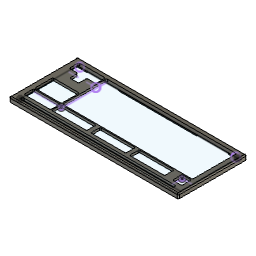
TKL assembled v2 (Autodesk Fusion 360 archive; units mm, degrees)
design "top attempt"
Autodesk Fusion 360 part; units mm, degrees
note: some values were not read from the file. Chosen so that the rebuilt part matches the saved one: which face or edge a step refers to. Set by a fixed rule: which sketch regions a step uses.
sketch "Sketch1" plane through (0, 0, 0) normal (1, 0, 0) x (0, 1, 0)
  line L0 (70, 20) -> (-80, 20)
  line L1 (-80, 20) -> (-80, 10)
  line L2 (-80, 10) -> (70, 10)
  line L3 (70, 10) -> (70, 20)
  constraint horizontal L0
  constraint vertical L1
  constraint horizontal L2
  constraint vertical L3
extrude "Extrude1" add sketch "Sketch1" along normal blind 185
move_face "OffsetFaces1" offset 185 1 faces at (0, -30, 13.3333)
sketch "Sketch2" plane through (0, 0, 20) normal (0, 0, 1) x (-1, 0, 0)
  line L0 (185, -70) -> (185, 80)
  line L1 (185, 80) -> (-185, 80)
  line L2 (-185, 80) -> (-185, -70)
  line L3 (-185, -70) -> (185, -70)
  line L4 (0, 0) -> (-110, 0)
  line L5 (0, 0) -> (175, 0)
  line L6 (0, 70) -> (0, 10)
  line L7 (0, 10) -> (0, -35)
  line L8 (175, 0) -> (175, -35)
  line L9 (175, -35) -> (-110, 70)
  line L10 (-110, -35) -> (-110, 70)
  line L11 (-110, 70) -> (175, 70)
  line L12 (175, 70) -> (175, -35)
  line L13 (-175, 70) -> (-116.5, 70)
  line L14 (-116.5, 70) -> (-116.5, 50.5)
  line L15 (-116.5, 50.5) -> (-175, 50.5)
  line L16 (-175, 50.5) -> (-175, 70)
  line L17 (-175, 50.5) -> (-155.5, 50.5)
  line L18 (-155.5, 50.5) -> (-155.5, 41.913)
  line L19 (-155.5, 50.5) -> (-155.5, 70)
  line L20 (-155.5, 41.913) -> (-136, 41.913)
  line L21 (-155.5, 70) -> (-136, 70)
  line L22 (-136, 70) -> (-136, 31)
  line L23 (-136, 31) -> (-155.5, 31)
  line L24 (-155.5, 31) -> (-155.5, 70)
  line L25 (-90, 70) -> (-90, -25)
  line L26 (-90, -25) -> (-110, -25)
  line L27 (-90, -25) -> (175, -25.0645)
  line L28 (-117.5, -25) -> (-175, -25)
  line L29 (-175, -25) -> (-175, 10)
  line L30 (-175, 10) -> (-117.5, 10)
  line L31 (-117.5, 10) -> (-117.5, -25)
  line L32 (-110, 8.1702) -> (-113, 8.1702)
  dimension "d4" = 110
  dimension "d5" = 175
  dimension "d8" = 60
  dimension "d9" = 45
  dimension "d12" = 19.5
  dimension "d13" = 19.5
  dimension "d14" = 19.5
  dimension "d15" = 39
  dimension "d16" = 95
  constraint coincident L4.start L5.start
  constraint horizontal L4
  constraint parallel L3 L5
  constraint perpendicular L4 L6
  constraint perpendicular L4 L7
  constraint perpendicular L5 L8
  constraint vertical L10
  constraint horizontal L11
  constraint vertical L12
  constraint perpendicular L13 L14
  constraint parallel L13 L15
  constraint parallel L14 L16
  constraint horizontal L13
  constraint horizontal L17
  constraint vertical L18
  constraint coincident L13 L19.end
  constraint perpendicular L13 L19
  constraint perpendicular L18 L20
  constraint horizontal L21
  constraint vertical L22
  constraint horizontal L23
  constraint vertical L24
  constraint coincident L11 L25.start
  constraint perpendicular L4 L25
  constraint coincident L10 L26.end
  constraint perpendicular L10 L26
  constraint coincident L8 L27.end
  constraint horizontal L28
  constraint vertical L29
  constraint horizontal L30
  constraint vertical L31
  constraint coincident L10 L32.start
  constraint perpendicular L31 L32
  measures "d4" distance of L4.start L4.end
  measures "d5" distance of L4.start L5.end
  measures "d8" distance of L6.start L6.end
  measures "d9" distance of L6.end L7.end
  measures "d12" distance of L13.start L15.end
  measures "d13" distance of L15.end L17.end
  measures "d14" distance of L18.end L20.end
  measures "d15" distance of L19.end L23.end
  measures "d16" distance of L25.start L25.end
sketch "Sketch3" plane through (0, 0, 0) normal (0, 0, 1) x (1, 0, 0)
extrude "Extrude2" add sketch "Sketch2" along normal blind 1 contours L28 L29 L30 L31
extrude "Extrude3" cut 1 faces at (136.6667, 13.3333, 21) along direction (0, 0, -1) blind 1
sketch "Sketch4" plane through (0, 0, 20) normal (0, 0, 1) x (-1, 0, 0)
  line L0 (185, -70) -> (185, 80)
  line L1 (185, 80) -> (-185, 80)
  line L2 (-185, 80) -> (-185, -70)
  line L3 (-185, -70) -> (185, -70)
  line L4 (-172.5, 0) -> (-172.5, -60)
  line L5 (172.5, 0) -> (172.5, 60)
  line L6 (-172.5, -60) -> (172.5, -60)
  line L7 (172.5, -60) -> (172.5, 60)
  line L8 (172.5, 60) -> (-172.5, 60)
  line L9 (-172.5, 60) -> (-172.5, -60)
  line L10 (0, -60) -> (0, 36)
  line L11 (-172.5, 36) -> (-172.5, -60)
  line L12 (-172.5, -60) -> (114.5, -60)
  line L13 (-172.5, -60) -> (111.5, -60)
  line L14 (-172.5, -60) -> (111.5, -60)
  line L15 (112, 36.5) -> (-172.5, 36.5)
  line L16 (-172.5, 36.5) -> (-172.5, -60)
  line L17 (172.5, -60) -> (115, -60)
  line L18 (172.5, -41) -> (172.5, -60)
  line L19 (153.5, -41) -> (134, -41)
  line L20 (134, -41) -> (134, -21)
  line L21 (134, -21) -> (153.5, -21)
  line L22 (153.5, -21) -> (153.5, -41)
  line L23 (172.5, 36) -> (172.5, -3)
  line L24 (172.5, 36) -> (172.5, -3)
  line L25 (172.5, -3) -> (112, -3)
  line L26 (-172.5, 60) -> (-152.5, 60)
  line L27 (-172.5, 40) -> (-172.5, 60)
  line L28 (172.5, 60) -> (114.5, 60)
  line L29 (114.5, 60) -> (114.5, 39)
  line L30 (114.5, 39) -> (172.5, 39)
  line L31 (172.5, 39) -> (172.5, 60)
  line L32 (-134.5, 60) -> (-58, 60)
  line L33 (-49, 60) -> (27.5, 60)
  line L34 (112, 39) -> (35.5, 39)
  line L35 (35.5, 39) -> (35.5, 60)
  line L36 (35.5, 60) -> (112, 60)
  line L37 (112, 60) -> (112, 39)
  line L38 (26.5, 55.7624) -> (26.5, 60.0294)
  line L39 (26.5, 60.0294) -> (-50, 60.0294)
  line L40 (-50, 60.0294) -> (-50, 39)
  line L41 (-50, 39) -> (26.5, 39)
  line L42 (26.5, 39) -> (26.5, 60.0294)
  line L43 (-58.5, 51.7468) -> (-58.5, 60)
  line L44 (-58.5, 60) -> (-135, 60)
  line L45 (-135, 60) -> (-135, 39)
  line L46 (-135, 39) -> (-58.5, 39)
  line L47 (-58.5, 39) -> (-58.5, 60)
  line L48 (114.5, -39) -> (172.5, -39)
  line L49 (115, -60) -> (112, -60)
  line L50 (112, -60) -> (112, 36.5)
  line L51 (114, 35) -> (115, 35)
  line L52 (115, 35) -> (114.5, 35)
  line L53 (114.5, 36) -> (114.5, -3)
  line L54 (114.5, -3) -> (114.5, -60)
  line L55 (114.5, 36) -> (114.5, 37)
  line L56 (114.5, 37) -> (114.5, 36.5)
  line L57 (117.4051, 36.5) -> (114.5, 36.5)
  line L58 (117.4051, 36.5) -> (172.5, 36.5)
  line L59 (112, 37) -> (112, 36.5)
  line L60 (-152.5, 60) -> (-152.5, 39)
  line L61 (-152.5, 39) -> (-172.5, 39)
  dimension "d21" = 172.5
  dimension "d22" = 172.5
  dimension "d24" = 96
  dimension "d26" = 284
  dimension "d27" = 57.5
  dimension "d28" = 19
  dimension "d29" = 19
  dimension "d31" = 39
  dimension "d32" = 20
  dimension "d33" = 20
  dimension "d37" = 76.5
  dimension "d39" = 4.267
  dimension "d41" = 76.5
  constraint horizontal L6
  constraint vertical L7
  constraint horizontal L8
  constraint vertical L9
  constraint midpoint L6 L10.start
  constraint vertical L11
  constraint horizontal L12
  constraint perpendicular L4 L13
  constraint horizontal L14
  constraint horizontal L15
  constraint vertical L16
  constraint perpendicular L7 L17
  constraint perpendicular L19 L20
  constraint parallel L19 L21
  constraint parallel L20 L22
  constraint vertical L24
  constraint horizontal L25
  constraint perpendicular L9 L26
  constraint horizontal L28
  constraint vertical L29
  constraint horizontal L30
  constraint vertical L31
  constraint coincident L8 L32.start
  constraint coincident L8 L33.start
  constraint perpendicular L34 L35
  constraint parallel L34 L36
  constraint parallel L35 L37
  constraint vertical L38
  constraint perpendicular L39 L40
  constraint parallel L39 L41
  constraint parallel L40 L42
  constraint perpendicular L38 L39
  constraint vertical L43
  constraint perpendicular L44 L45
  constraint parallel L44 L46
  constraint parallel L45 L47
  constraint coincident L8 L44.end
  constraint coincident L7 L48.end
  constraint perpendicular L7 L48
  constraint coincident L6 L49.end
  constraint perpendicular L15 L50
  constraint coincident L25.end L50
  constraint perpendicular L50 L51
  constraint midpoint L51 L52.end
  constraint parallel L51 L52
  constraint coincident L25 L53.end
  constraint perpendicular L25 L53
  constraint parallel L53 L55
  constraint midpoint L55 L56.end
  constraint parallel L55 L56
  constraint perpendicular L55 L57
  constraint coincident L5 L58.end
  constraint coincident L7 L58.end
  constraint perpendicular L15 L59
  constraint perpendicular L26 L60
  constraint coincident L9 L61.end
  constraint perpendicular L9 L61
  constraint coincident L48.start L54
  measures "d21" distance of origin L4.start
  measures "d22" distance of origin L5.start
  measures "d24" distance of L10.start L10.end
  measures "d26" distance of L4.end L13.end
  measures "d27" distance of L6.end L17.end
  measures "d28" distance of L6.end L18.start
  measures "d29" distance of L18.start L19.start
  measures "d31" distance of L23.start L23.end
  measures "d32" distance of L8.end L26.end
  measures "d33" distance of L8.end L27.start
  measures "d37" distance of L34.start L34.end
  measures "d39" distance of L38.start L38.end
  measures "d41" distance of L43.end L44.end
extrude "Extrude4" cut sketch "Sketch4" against normal blind 20 contours L4 L6 L9 L11 L12 L13 L14 L15 L16 L50 | L8 L9 L26 L27 L60 L61 | L6 L7 L17 L18 L19 L20 L22 L48 L49 L54 | L5 L7 L23 L24 L25 L53 L55 L57 L58 | L8 L32 L43 L44 L45 L46 L47 | L19 L20 L22 L48 | L20 L21 L22 L48 | L8 L33 L38 L40 L41 L42 | L5 L7 L8 L28 L29 L30 L31 | L8 L34 L35 L36 L37
fillet "Fillet1" radius 2 2 edges at (172.5, 60, 15) (172.5, -36.5, 15)
fillet "Fillet2" radius 2 4 edges at (-35.5, -60, 15) (-35.5, -39, 15) (-112, -39, 15) (-112, -60, 15)
fillet "Fillet3" radius 2 4 edges at (-26.5, -60, 15) (-26.5, -39, 15) (50, -39, 15) (50, -60, 15)
fillet "Fillet4" radius 2 4 edges at (-114.5, -60, 15) (-114.5, -39, 15) (-172.5, -39, 15) (-172.5, -60, 15)
fillet "Fillet5" radius 2 1 edges at (-172.5, 3, 15)
fillet "Fillet6" radius 2 3 edges at (-172.5, 60, 15) (-153.5, 21, 15) (-134, 21, 15)
fillet "Fillet7" radius 2 4 edges at (135, -60, 15) (58.5, -60, 15) (58.5, -39, 15) (135, -39, 15)
fillet "Fillet8" radius 2 1 edges at (172.5, -60, 15)
fillet "Fillet9" radius 2.5 4 edges at (0, 70, 20) (185, -5, 20) (0, -80, 20) (-185, -5, 20)
sketch "Sketch5" plane through (0, 0, 0) normal (0, 0, 1) x (1, 0, 0)
  arc A0 (-150, 65) -> (-155, 60) centre (-150, 60) ccw
  line L0 (-150, 65) -> (-90, 65)
  arc A1 (-85, 60) -> (-90, 65) centre (-90, 60) ccw
  arc A2 (155, 60) -> (150, 65) centre (150, 60) ccw
  line L1 (150, 65) -> (90, 65)
  arc A3 (90, 65) -> (85, 60) centre (90, 60) ccw
  line L2 (-155, 60) -> (-85, 60)
  line L3 (85, 60) -> (155, 60)
  arc A4 (150, -70) -> (155, -65) centre (150, -65) ccw
  line L4 (150, -70) -> (90, -70)
  arc A5 (85, -65) -> (90, -70) centre (90, -65) ccw
  line L5 (85, -65) -> (155, -65)
  line L6 (0, -70) -> (30, -70)
  line L7 (0, -70) -> (-30, -70)
  arc A6 (30, -70) -> (35, -65) centre (30, -65) ccw
  arc A7 (-35, -65) -> (-30, -70) centre (-30, -65) ccw
  line L8 (-35, -65) -> (35, -65)
  line L9 (-150, -65) -> (-155, -65)
  arc A8 (-155, -65) -> (-150, -70) centre (-150, -65) ccw
  line L10 (-150, -70) -> (-90, -70)
  arc A9 (-90, -70) -> (-85, -65) centre (-90, -65) ccw
  line L11 (-150, -65) -> (-85, -65)
  line L12 (-176, -65) -> (175, -65)
  line L13 (175, -65) -> (175, 60)
  line L14 (175, 60) -> (-176, 60)
  line L15 (-176, 60) -> (-176, -65)
  dimension "d62" = 60
  dimension "d63" = 60
  dimension "d64" = 60
  dimension "d65" = 30
  dimension "d66" = 30
  constraint horizontal L0
  constraint horizontal L1
  constraint parallel L0 L2
  constraint parallel L1 L3
  constraint horizontal L4
  constraint horizontal L5
  constraint parallel L5 L6
  constraint parallel L6 L7
  constraint horizontal L8
  constraint parallel L8 L9
  constraint coincident L9.start A8.centre
  constraint tangent A8 L10
  constraint horizontal L10
  constraint parallel L9 L11
  constraint horizontal L12
  constraint vertical L13
  constraint horizontal L14
  constraint vertical L15
  measures "d62" distance of A0.start L0.end
  measures "d63" distance of A2.end L1.end
  measures "d64" distance of A4.start L4.end
  measures "d65" distance of L6.start L6.end
  measures "d66" distance of L6.start L7.end
move_body "Move1" bodies 1 to x (1, 0, 0) y (0, 1, 0) z (0, 0, 1) at (0, 0, -10)
extrude "Extrude5" cut sketch "Sketch5" along normal blind 2.5
sketch "Sketch6" plane through (0, 0, 2.5) normal (0, 0, -1) x (1, 0, 0)
  arc A0 (-172.5, -58) -> (-170.5, -60) centre (-170.5, -58) ccw
  line L0 (-172.5, -58) -> (-172.5, -39)
  line L1 (-153.5, -39) -> (-153.5, -23)
  arc A1 (-151.5, -21) -> (-153.5, -23) centre (-151.5, -23) ccw
  line L2 (-151.5, -21) -> (-136, -21)
  arc A2 (-134, -23) -> (-136, -21) centre (-136, -23) ccw
  line L3 (-134, -23) -> (-134, -39)
  line L4 (-114.5, -60) -> (-155, -60)
  arc A3 (-155, -60) -> (-150, -65) centre (-150, -60) ccw
  line L5 (-150, -65) -> (-90, -65)
  arc A4 (-90, -65) -> (-85, -60) centre (-90, -60) ccw
  line L6 (-85, -60) -> (-112, -60)
  line L7 (-112, 36.5) -> (170.5, 36.5)
  arc A5 (172.5, 34.5) -> (170.5, 36.5) centre (170.5, 34.5) ccw
  line L8 (172.5, 34.5) -> (172.5, -58)
  arc A6 (170.5, -60) -> (172.5, -58) centre (170.5, -58) ccw
  line L9 (170.5, -60) -> (175, -60)
  line L10 (175, -60) -> (175, 65)
  line L11 (175, 65) -> (155, 65)
  arc A7 (155, 65) -> (150, 70) centre (150, 65) ccw
  line L12 (150, 70) -> (90, 70)
  arc A8 (90, 70) -> (85, 65) centre (90, 65) ccw
  line L13 (85, 65) -> (35, 65)
  arc A9 (35, 65) -> (30, 70) centre (30, 65) ccw
  line L14 (30, 70) -> (-30, 70)
  arc A10 (-30, 70) -> (-35, 65) centre (-30, 65) ccw
  line L15 (-35, 65) -> (-85, 65)
  arc A11 (-85, 65) -> (-90, 70) centre (-90, 65) ccw
  line L16 (-90, 70) -> (-150, 70)
  arc A12 (-150, 70) -> (-155, 65) centre (-150, 65) ccw
  line L17 (-155, 65) -> (-176, 65)
  line L18 (-176, 65) -> (-176, -60)
  line L19 (-176, -60) -> (-170.5, -60)
  line L20 (152.5, 60) -> (170.5, 60)
  arc A13 (172.5, 58) -> (170.5, 60) centre (170.5, 58) ccw
  line L21 (172.5, 58) -> (172.5, 39)
  arc A14 (133, 39) -> (135, 41) centre (133, 41) ccw
  line L22 (133, 39) -> (60.5, 39)
  arc A15 (58.5, 41) -> (60.5, 39) centre (60.5, 41) ccw
  line L23 (58.5, 41) -> (58.5, 58)
  arc A16 (60.5, 60) -> (58.5, 58) centre (60.5, 58) ccw
  line L24 (60.5, 60) -> (133, 60)
  arc A17 (135, 58) -> (133, 60) centre (133, 58) ccw
  line L25 (135, 58) -> (135, 41)
  line L26 (-114.5, -3) -> (-170.5, -3)
  arc A18 (-172.5, -1) -> (-170.5, -3) centre (-170.5, -1) ccw
  line L27 (-172.5, -1) -> (-172.5, 36.5)
  arc A19 (-116.5, 39) -> (-114.5, 41) centre (-116.5, 41) ccw
  line L28 (-116.5, 39) -> (-170.5, 39)
  arc A20 (-172.5, 41) -> (-170.5, 39) centre (-170.5, 41) ccw
  line L29 (-172.5, 41) -> (-172.5, 58)
  arc A21 (-170.5, 60) -> (-172.5, 58) centre (-170.5, 58) ccw
  line L30 (-170.5, 60) -> (-116.5, 60)
  arc A22 (-114.5, 58) -> (-116.5, 60) centre (-116.5, 58) ccw
  line L31 (-114.5, 58) -> (-114.5, 41)
  arc A23 (50, 58) -> (48, 60) centre (48, 58) ccw
  line L32 (50, 58) -> (50, 41)
  arc A24 (48, 39) -> (50, 41) centre (48, 41) ccw
  line L33 (48, 39) -> (-24.5, 39)
  arc A25 (-26.5, 41) -> (-24.5, 39) centre (-24.5, 41) ccw
  line L34 (-26.5, 41) -> (-26.5, 58)
  arc A26 (-24.5, 60) -> (-26.5, 58) centre (-24.5, 58) ccw
  line L35 (-24.5, 60) -> (48, 60)
  arc A27 (-37.5, 39) -> (-35.5, 41) centre (-37.5, 41) ccw
  line L36 (-37.5, 39) -> (-110, 39)
  arc A28 (-112, 41) -> (-110, 39) centre (-110, 41) ccw
  line L37 (-112, 41) -> (-112, 58)
  arc A29 (-110, 60) -> (-112, 58) centre (-110, 58) ccw
  line L38 (-110, 60) -> (-37.5, 60)
  arc A30 (-35.5, 58) -> (-37.5, 60) centre (-37.5, 58) ccw
  line L39 (-35.5, 58) -> (-35.5, 41)
  line L40 (-176, 65) -> (175, 65)
  line L41 (175, 65) -> (175, -60)
  line L42 (175, -60) -> (-176, -60)
  line L43 (-176, -60) -> (-176, 65)
  line L44 (-114.5, 36.5) -> (-114.5, -3)
  line L45 (-172.5, 36.5) -> (-114.5, 36.5)
  line L46 (172.5, 39) -> (152.5, 39)
  line L47 (152.5, 39) -> (152.5, 60)
  line L48 (-172.5, -39) -> (-153.5, -39)
  line L49 (-134, -39) -> (-114.5, -39)
  line L50 (-114.5, -39) -> (-114.5, -60)
  line L51 (-112, -60) -> (-112, 36.5)
  constraint horizontal L40
  constraint vertical L41
  constraint horizontal L42
  constraint vertical L43
  constraint coincident L9.end L10.start
  constraint coincident L17.end L18.start
sketch "Sketch7" plane through (0, 0, 0) normal (0, 0, 1) x (1, 0, 0)
  line L0 (-176, -65) -> (175, -65)
  line L1 (175, -65) -> (175, 60)
  line L2 (175, 60) -> (-176, 60)
  line L3 (-176, 60) -> (-176, -65)
  constraint horizontal L0
  constraint vertical L1
  constraint horizontal L2
  constraint vertical L3
extrude "Extrude6" cut sketch "Sketch7" along normal blind 5
sketch "Sketch8" plane through (0, 0, 10) normal (0, 0, 1) x (-1, 0, 0)
  line L0 (-172.5, 39) -> (-172.5, 58)
  arc A0 (-170.5, 60) -> (-172.5, 58) centre (-170.5, 58) ccw
  line L1 (-170.5, 60) -> (-152.5, 60)
  line L2 (112, -60) -> (-170.5, -60)
  arc A1 (-172.5, -58) -> (-170.5, -60) centre (-170.5, -58) ccw
  line L3 (-172.5, -58) -> (-172.5, 34.5)
  arc A2 (-170.5, 36.5) -> (-172.5, 34.5) centre (-170.5, 34.5) ccw
  line L4 (-170.5, 36.5) -> (112, 36.5)
  line L5 (35.5, 41) -> (35.5, 58)
  arc A3 (37.5, 60) -> (35.5, 58) centre (37.5, 58) ccw
  line L6 (37.5, 60) -> (110, 60)
  arc A4 (112, 58) -> (110, 60) centre (110, 58) ccw
  line L7 (112, 58) -> (112, 41)
  arc A5 (110, 39) -> (112, 41) centre (110, 41) ccw
  line L8 (110, 39) -> (37.5, 39)
  arc A6 (35.5, 41) -> (37.5, 39) centre (37.5, 41) ccw
  line L9 (172.5, 36.5) -> (172.5, -1)
  arc A7 (170.5, -3) -> (172.5, -1) centre (170.5, -1) ccw
  line L10 (170.5, -3) -> (114.5, -3)
  line L11 (-133, 60) -> (-60.5, 60)
  arc A8 (-58.5, 58) -> (-60.5, 60) centre (-60.5, 58) ccw
  line L12 (-58.5, 58) -> (-58.5, 41)
  arc A9 (-60.5, 39) -> (-58.5, 41) centre (-60.5, 41) ccw
  line L13 (-60.5, 39) -> (-133, 39)
  arc A10 (-135, 41) -> (-133, 39) centre (-133, 41) ccw
  line L14 (-135, 41) -> (-135, 58)
  arc A11 (-133, 60) -> (-135, 58) centre (-133, 58) ccw
  line L15 (-50, 41) -> (-50, 58)
  arc A12 (-48, 60) -> (-50, 58) centre (-48, 58) ccw
  line L16 (-48, 60) -> (24.5, 60)
  arc A13 (26.5, 58) -> (24.5, 60) centre (24.5, 58) ccw
  line L17 (26.5, 58) -> (26.5, 41)
  arc A14 (24.5, 39) -> (26.5, 41) centre (24.5, 41) ccw
  line L18 (24.5, 39) -> (-48, 39)
  arc A15 (-50, 41) -> (-48, 39) centre (-48, 41) ccw
  line L19 (116.5, 60) -> (170.5, 60)
  arc A16 (172.5, 58) -> (170.5, 60) centre (170.5, 58) ccw
  line L20 (172.5, 58) -> (172.5, 41)
  arc A17 (170.5, 39) -> (172.5, 41) centre (170.5, 41) ccw
  line L21 (170.5, 39) -> (116.5, 39)
  arc A18 (114.5, 41) -> (116.5, 39) centre (116.5, 41) ccw
  line L22 (114.5, 41) -> (114.5, 58)
  arc A19 (116.5, 60) -> (114.5, 58) centre (116.5, 58) ccw
  line L23 (172.5, -39) -> (172.5, -58)
  arc A20 (170.5, -60) -> (172.5, -58) centre (170.5, -58) ccw
  line L24 (170.5, -60) -> (114.5, -60)
  line L25 (134, -39) -> (134, -23)
  arc A21 (136, -21) -> (134, -23) centre (136, -23) ccw
  line L26 (136, -21) -> (151.5, -21)
  arc A22 (153.5, -23) -> (151.5, -21) centre (151.5, -23) ccw
  line L27 (153.5, -23) -> (153.5, -39)
  line L28 (182.5, -67.5) -> (182.5, 77.5)
  line L29 (182.5, 77.5) -> (-182.5, 77.5)
  line L30 (-182.5, 77.5) -> (-182.5, -67.5)
  line L31 (-182.5, -67.5) -> (182.5, -67.5)
  arc A23 (-165.0446, 72.9997) -> (-165, 67) centre (-165, 70) ccw
  arc A24 (165, 67) -> (165, 73) centre (165, 70) ccw
  line L32 (-165.0446, 72.9997) -> (165, 73)
  line L33 (-165, 67) -> (165, 67)
  line L34 (114.5, -3) -> (114.5, 36.5)
  line L35 (114.5, 36.5) -> (172.5, 36.5)
  line L36 (153.5, -39) -> (172.5, -39)
  line L37 (114.5, -60) -> (114.5, -39)
  line L38 (114.5, -39) -> (134, -39)
  line L39 (-152.5, 39) -> (-172.5, 39)
  line L40 (-152.5, 60) -> (-152.5, 39)
  line L41 (112, 36.5) -> (112, -60)
  constraint tangent A24 L32
  constraint tangent A24 L33
extrude "Extrude7" cut sketch "Sketch8" against normal blind 5 contours A23 A24 L32 L33
fillet "Fillet10" radius 2.5 8 edges at (184.2678, -79.2678, 9.2678) (185, -80, 3.75) (185, 70, 3.75) (184.2678, 69.2678, 9.2678) (-185, 70, 3.75) (-184.2678, 69.2678, 9.2678) (-184.2678, -79.2678, 9.2678) (-185, -80, 3.75)
fillet "Fillet11" radius 2.5 3 edges at (152.5, -39, 7.5) (172.5, -39, 7.5) (152.5, -60, 7.5)
fillet "Fillet12" radius 2.5 3 edges at (-172.5, -36.5, 7.5) (-114.5, -36.5, 7.5) (-114.5, 3, 7.5)
fillet "Fillet13" radius 2.5 3 edges at (-114.5, 60, 7.5) (-134, 39, 7.5) (-153.5, 39, 7.5)
fillet "Fillet14" radius 2.5 1 edges at (-172.5, 39, 7.5)
fillet "Fillet15" radius 2.5 2 edges at (-112, 60, 7.5) (-112, -36.5, 7.5)
fillet "Fillet16" radius 2.5 1 edges at (-114.5, 39, 7.5)
